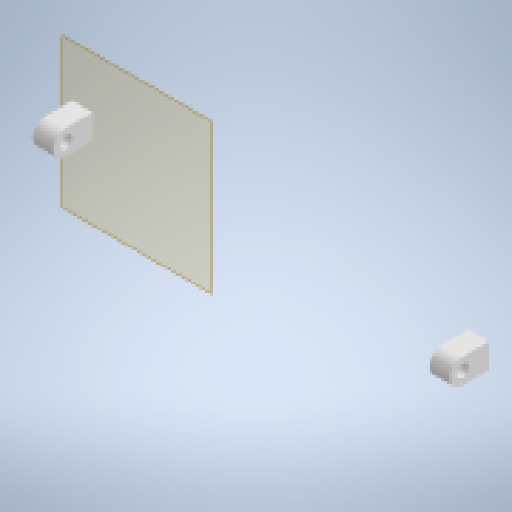
# Autodesk Inventor part: BEVEL_SHAFT
Saved by Autodesk Inventor 2024 (Build 280153000, 153)
## iProperties
Created: 2024-04-16
Part Number: BEVEL_SHAFT
Material: Generic
Document SubType Name: Modeling
Designer: teeta
Density: 1 g/cm^3
Appearance: Default
Author: teeta
Autodesk Inventor part; units mm, degrees
ref_plane "YZ Plane" through (0, 0, 0) normal (1, 0, 0) x (0, 1, 0)
ref_plane "XZ Plane" through (0, 0, 0) normal (0, 1, 0) x (-1, 0, 0)
ref_plane "XY Plane" through (0, 0, 0) normal (0, 0, 1) x (1, 0, 0)
ref_plane "Work Plane1" through (0, 0, 0) normal (0, 0, 1) x (1, 0, 0)
sketch "Sketch1" plane through (0, 0, 0) normal (0, 0, 1) x (1, 0, 0)
  line L0 (-134.0646, -12.3024) -> (-92.7896, -12.3024)
  line L1 (-92.7896, -12.3024) -> (-92.7896, 37.6976)
  line L2 (-92.7896, 37.6976) -> (-134.0646, 37.6976)
  line L3 (-134.0646, 37.6976) -> (-134.0646, -12.3024)
  line L4 (710.3854, 1102.2976) -> (710.3854, -142.1524) projected
  line L5 (707.2104, -138.9774) -> (-130.8896, -138.9774) projected
  line L6 (288.1604, -138.9774) -> (288.1604, 728.5141) construction
  line L7 (710.3854, -12.3024) -> (669.1104, -12.3024)
  line L8 (669.1104, -12.3024) -> (669.1104, 37.6976)
  line L9 (669.1104, 37.6976) -> (710.3854, 37.6976)
  line L10 (710.3854, 37.6976) -> (710.3854, -12.3024)
  point P0 (0, 0)
  constraints: 18 end point, 4 symmetric about line, 2 parallel, 1 horizontal, 1 midpoint, 1 perpendicular, 1 vertical
extrude "Extrusion1" add sketch "Sketch1" along normal blind 80
sketch "Sketch2" plane through (710.3854, -12.3024, 0) normal (1, 0, 0) x (0, 0, -1)
  circle A0 centre (-53.553, 25) radius 12.5
  line L0 (0, 50) -> (-80, 50) projected
  point P0 (0, 12.3024)
  dimension "d2" = 25
  dimension "d3" = 25
  constraints: 1 centre point
  measures "d2" distance from line of L0 A0.centre
  measures "d3" diameter of A0
extrude "Extrusion2" cut sketch "Sketch2" against normal through all
fillet "Fillet1" radius 25 4 edges at (689.7479, -12.3024, 80) (689.7479, 37.6976, 80) (-113.4271, -12.3024, 80) (-113.4271, 37.6976, 80)
body "Solid1"
